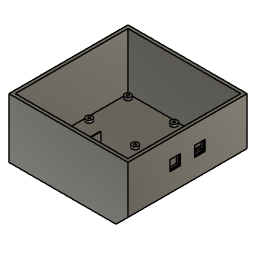
WeatherBox (Autodesk Fusion 360 design; units mm, degrees)
Autodesk Fusion 360 part; units mm, degrees
note: some values were not read from the file. Set by a fixed rule: which face or edge a step refers to.
sketch "Enclosure" plane through (0, 0, 0) normal (0, 0, 1) x (1, 0, 0)
  line L0 (0, 0) -> (150, 0)
  line L1 (150, 0) -> (150, 150)
  line L2 (150, 150) -> (0, 150)
  line L3 (0, 150) -> (0, 0)
  dimension "d1" = 150
  dimension "d2" = 150
  constraint horizontal L0
  constraint vertical L1
  constraint horizontal L2
  constraint vertical L3
  constraint coincident L0.start L3.end
  measures "d1" distance of L0.start L0.end
  measures "d2" distance of L0.start L2.end
extrude "Extrude1" add sketch "Enclosure" along normal blind 75 makes body 1
chamfer "Chamfer1" distance 15 angle 45 1 edges at (150, 75, 0) on bodies 1
shell "Shell1" thickness 4 removed faces 1 at (50, 100, 75) on bodies 1
sketch "Pi Mount" plane through (0, 0, 4) normal (0, 0, 1) x (-1, 0, 0)
  line L0 (-4, -146) -> (-4, -4)
  line L1 (-4, -4) -> (-133.3431, -4)
  line L2 (-133.3431, -146) -> (-4, -146)
  circle A0 centre (-9, -141) radius 4
  line L3 (-133.3431, -4) -> (-133.3431, -146)
  dimension "d13" = 8
  dimension "d39" = 5
  dimension "d40" = 5
  measures "d13" diameter of A0
  measures "d39" distance of L2 A0.centre
  measures "d40" distance of L0 A0.centre
extrude "Extrude2" add sketch "Pi Mount" along normal blind 3.1 contours A0 bodies 1
hole "Hole2" at (9, 141, 7.1) direction (0, 0, -1) diameter 2.9 depth 3.1 tip angle 180 bodies 1
pattern_linear "R-Pattern1" count 2 spacing 58 along (1, 0, 0) count 2 spacing 49 along (0, -1, 0) of "Extrude2", "Hole2"
sketch "Camera Holes" plane through (150, 0, 0) normal (1, 0, 0) x (0, 1, 0)
  line L0 (150, 15) -> (150, 75)
  line L1 (150, 75) -> (0, 75)
  line L2 (0, 75) -> (0, 15)
  line L3 (65, 39.45) -> (53.9, 39.45)
  line L4 (53.9, 39.45) -> (53.9, 50.55)
  line L5 (53.9, 50.55) -> (65, 50.55)
  line L6 (65, 50.55) -> (65, 39.45)
  line L7 (65, 39.45) -> (53.9, 50.55) construction
  line L8 (53.9, 39.45) -> (65, 50.55) construction
  line L9 (0, 45) -> (150, 45) construction
  line L10 (75, 75) -> (75, 0) construction
  line L11 (96.1, 39.45) -> (85, 50.55) construction
  line L12 (85, 39.45) -> (96.1, 50.55) construction
  line L13 (85, 39.45) -> (85, 50.55)
  line L14 (85, 50.55) -> (96.1, 50.55)
  line L15 (96.1, 50.55) -> (96.1, 39.45)
  line L16 (96.1, 39.45) -> (85, 39.45)
  line L17 (66, 38.45) -> (52.9, 38.45)
  line L18 (52.9, 38.45) -> (52.9, 51.55)
  line L19 (52.9, 51.55) -> (66, 51.55)
  line L20 (66, 51.55) -> (66, 38.45)
  line L21 (97.1, 38.45) -> (84, 38.45)
  line L22 (84, 38.45) -> (84, 51.55)
  line L23 (84, 51.55) -> (97.1, 51.55)
  line L24 (97.1, 51.55) -> (97.1, 38.45)
  line L25 (0, 15) -> (150, 15)
  point P0 (59.45, 45)
  point P1 (90.55, 45)
  dimension "d92" = 11.1
  dimension "d93" = 11.1
  dimension "d168" = 11.1
  dimension "d169" = 11.1
  dimension "d170" = 20
  dimension "d177" = -1
  dimension "d178" = -1
  constraint horizontal L3
  constraint perpendicular L3 L4
  constraint parallel L3 L5
  constraint parallel L4 L6
  constraint coincident L7 P0
  constraint coincident L8 P0
  constraint midpoint L2 L9.start
  constraint midpoint L0 L9.end
  constraint coincident P0 L9
  constraint midpoint L1 L10.start
  constraint horizontal L16
  constraint perpendicular L13 L16
  constraint parallel L14 L16
  constraint parallel L13 L15
  constraint coincident P1 L11
  constraint coincident P1 L12
  constraint symmetric L6 L10 L13
  constraint collinear L19 L23
  measures "d92" distance of L4.end L5.end
  measures "d93" distance of L3.end L4.end
  measures "d168" distance of L12.end L11.end
  measures "d169" distance of L12.start L11.end
  measures "d170" distance of L6 L13
extrude "Extrude6" cut sketch "Camera Holes" against normal up to surface (4 mm away) contours L3 L4 L5 L6 | L13 L14 L15 L16 bodies 1
extrude "Extrude10" cut sketch "Camera Holes" against normal blind 1.5375 contours L17 L18 L19 L20 | L21 L22 L23 L24 bodies 1
sketch "Camera Mounts" plane through (146, 0, 0) normal (-1, 0, 0) x (0, -1, 0)
  line L0 (-65, 39.45) -> (-65, 50.55)
  line L1 (-65, 50.55) -> (-53.9, 50.55)
  line L2 (-53.9, 50.55) -> (-53.9, 39.45)
  line L3 (-53.9, 39.45) -> (-65, 39.45)
  line L4 (-4, 16.6569) -> (-4, 75)
  line L5 (-4, 75) -> (-146, 75)
  line L6 (-146, 75) -> (-146, 16.6569)
  line L7 (-69.95, 57.6) -> (-48.95, 57.6) construction
  line L8 (-48.95, 57.6) -> (-48.95, 45.1) construction
  line L9 (-48.95, 45.1) -> (-69.95, 45.1) construction
  line L10 (-69.95, 45.1) -> (-69.95, 57.6) construction
  line L11 (-59.45, 50.55) -> (-59.45, 45) construction
  line L12 (-59.45, 45) -> (-53.9, 45) construction
  line L13 (-85, 39.45) -> (-96.1, 39.45)
  line L14 (-96.1, 39.45) -> (-96.1, 50.55)
  line L15 (-96.1, 50.55) -> (-85, 50.55)
  line L16 (-85, 50.55) -> (-85, 39.45)
  line L17 (-101.05, 57.6) -> (-80.05, 57.6) construction
  line L18 (-101.05, 45.1) -> (-101.05, 57.6) construction
  line L19 (-80.05, 45.1) -> (-101.05, 45.1) construction
  line L20 (-80.05, 57.6) -> (-80.05, 45.1) construction
  line L21 (-85, 45) -> (-90.55, 45) construction
  line L22 (-90.55, 45) -> (-90.55, 50.55) construction
  line L23 (-146, 16.6569) -> (-4, 16.6569)
  dimension "d131" = 21
  dimension "d132" = 12.5
  dimension "d173" = 21
  dimension "d174" = 12.5
  dimension "d176" = 0.1
  constraint horizontal L7
  constraint vertical L8
  constraint horizontal L9
  constraint vertical L10
  constraint midpoint L1 L11.start
  constraint perpendicular L1 L11
  constraint midpoint L2 L12.end
  constraint perpendicular L2 L12
  constraint horizontal L17
  constraint vertical L20
  constraint horizontal L19
  constraint vertical L18
  constraint midpoint L16 L21.start
  constraint midpoint L15 L22.end
  constraint perpendicular L15 L22
  constraint symmetric L18 L20 L22
  constraint collinear L9 L19
  measures "d131" distance of L7.start L7.end
  measures "d132" distance of L7.start L9.end
  measures "d173" distance of L17.start L17.end
  measures "d174" distance of L17.start L18.start
  measures "d176" distance of L19 L21
hole "Hole7" at (146, 48.95, 57.6) at (146, 69.95, 45.1) at (146, 80.05, 57.6) at (146, 101.05, 57.6) at (146, 101.05, 45.1) at (146, 80.05, 45.1) at (146, 69.95, 57.6) at (146, 48.95, 45.1) direction (1, 0, 0) diameter 2.9 depth 2 tip angle 180 bodies 1
sketch "Camera Posts" plane through (146, 0, 0) normal (-1, 0, 0) x (0, -1, 0)
  circle A0 centre (-101.05, 45.1) radius 1.45
  circle A1 centre (-80.05, 57.6) radius 1.45
  circle A2 centre (-48.95, 45.1) radius 1.45
  circle A3 centre (-69.95, 57.6) radius 1.45
  circle A4 centre (-48.95, 57.6) radius 1.45
  circle A5 centre (-69.95, 45.1) radius 1.45
  circle A6 centre (-101.05, 57.6) radius 1.45
  circle A7 centre (-80.05, 45.1) radius 1.45
  line L0 (-65, 39.45) -> (-65, 50.55)
  line L1 (-65, 50.55) -> (-53.9, 50.55)
  line L2 (-53.9, 50.55) -> (-53.9, 39.45)
  line L3 (-53.9, 39.45) -> (-65, 39.45)
  line L4 (-85, 39.45) -> (-96.1, 39.45)
  line L5 (-96.1, 39.45) -> (-96.1, 50.55)
  line L6 (-96.1, 50.55) -> (-85, 50.55)
  line L7 (-85, 50.55) -> (-85, 39.45)
  line L8 (-4, 16.6569) -> (-4, 75)
  line L9 (-4, 75) -> (-146, 75)
  line L10 (-146, 75) -> (-146, 16.6569)
  circle A8 centre (-101.05, 57.6) radius 3.95
  circle A9 centre (-80.05, 57.6) radius 3.95
  circle A10 centre (-101.05, 45.1) radius 3.95
  circle A11 centre (-80.05, 45.1) radius 3.95
  circle A12 centre (-69.95, 57.6) radius 3.95
  circle A13 centre (-48.95, 57.6) radius 3.95
  circle A14 centre (-48.95, 45.1) radius 3.95
  circle A15 centre (-69.95, 45.1) radius 3.95
  line L11 (-146, 16.6569) -> (-4, 16.6569)
  dimension "d193" = 2.5
  constraint equal A8 A10
  constraint equal A8 A11
  constraint equal A8 A9
  constraint equal A8 A12
  constraint equal A8 A15
  constraint equal A8 A14
  constraint equal A8 A13
extrude "Extrude11" add sketch "Camera Posts" along normal blind 7 contours A8 | A9 | A10 | A11 | A12 | A13 | A14 | A15 bodies 1
sketch "SPS30 Mount" plane through (0, 4, 0) normal (0, 1, 0) x (-1, 0, 0)
  line L0 (-4, 75) -> (-146, 75)
  line L1 (-133.3431, 4) -> (-4, 4)
  line L2 (-130, 64) -> (-82.45, 64)
  line L3 (-82.45, 64) -> (-82.45, 16.45)
  line L4 (-82.45, 16.45) -> (-130, 16.45)
  line L5 (-130, 16.45) -> (-130, 64)
  line L6 (-81.45, 15.45) -> (-131, 15.45)
  line L7 (-131, 15.45) -> (-131, 65)
  line L8 (-131, 65) -> (-81.45, 65)
  line L9 (-81.45, 65) -> (-81.45, 15.45)
  line L10 (-102.45, 16.45) -> (-102.45, 15.45)
  line L11 (-130, 16.45) -> (-130, 15.45)
  line L12 (-84.45, 64) -> (-84.45, 65)
  line L13 (-125, 64) -> (-125, 65)
  line L14 (-139.7177, 40.225) -> (-2.7177, 40.225) construction
  line L15 (-106.225, 64) -> (-106.225, 16.45) construction
  line L16 (-130, 40.225) -> (-82.45, 40.225) construction
  line L17 (-4, 4) -> (-4, 75)
  line L18 (-146, 75) -> (-146, 16.6569)
  line L19 (-99.45, 64) -> (-99.45, 75)
  line L20 (-99.45, 75) -> (-98.45, 75)
  line L21 (-98.45, 75) -> (-98.45, 64)
  line L22 (-99.45, 64) -> (-98.45, 64)
  line L23 (-77.45, 40.225) -> (-135, 40.225) construction
  circle A0 centre (-77.45, 40.225) radius 2.35
  circle A1 centre (-135, 40.225) radius 2.35
  circle A2 centre (-135, 40.225) radius 4.85
  circle A3 centre (-77.45, 40.225) radius 4.85
  line L24 (-77.45, 45.075) -> (-135, 45.075)
  line L25 (-135, 35.375) -> (-77.45, 35.375)
  line L26 (-146, 16.6569) -> (-133.3431, 4)
  dimension "d118" = 47.55
  dimension "d119" = 47.55
  dimension "d121" = -1
  dimension "d122" = 20
  dimension "d124" = 2
  dimension "d125" = 5
  dimension "d143" = 16
  dimension "d182" = 15
  dimension "d184" = 10
  dimension "d203" = 1
  dimension "d225" = 57.55
  dimension "d229" = 4.7
  dimension "d230" = 4.7
  dimension "d231" = 2.5
  dimension "d232" = 2.5
  constraint horizontal L2
  constraint vertical L3
  constraint horizontal L4
  constraint vertical L5
  constraint coincident L4 L10.start
  constraint coincident L6 L10.end
  constraint perpendicular L6 L10
  constraint coincident L6 L11.end
  constraint perpendicular L6 L11
  constraint coincident L2 L12.start
  constraint coincident L8 L12.end
  constraint perpendicular L8 L12
  constraint coincident L2 L13.start
  constraint coincident L8 L13.end
  constraint perpendicular L8 L13
  constraint midpoint L2 L15.start
  constraint midpoint L4 L15.end
  constraint midpoint L5 L16.start
  constraint midpoint L3 L16.end
  constraint collinear L14 L16
  constraint vertical L19
  constraint horizontal L20
  constraint vertical L21
  constraint coincident L0 L19.end
  constraint coincident L2 L19.start
  constraint coincident L2 L21.end
  constraint coincident L14 L23.start
  constraint perpendicular L15 L23
  constraint midpoint L15 L23
  constraint coincident L23.start A0.centre
  constraint coincident L23.end A1.centre
  constraint coincident A3 L24.start
  constraint coincident A2 L24.end
  constraint coincident A2 L25.start
  constraint coincident A3 L25.end
  constraint tangent A3 L24
  constraint tangent A3 L25
  constraint tangent A2 L25
  constraint tangent A2 L24
  measures "d118" distance of L2.start L4.end
  measures "d119" distance of L2.start L2.end
  measures "d122" distance of L3 L10
  measures "d124" distance of L3 L12
  measures "d125" distance of L5 L13
  measures "d143" distance of L3 L21
  measures "d182" distance of L7 L18
  measures "d184" distance of L0 L8
  measures "d203" distance of L21.end L19.start
  measures "d225" distance of L23.start L23.end
  measures "d229" diameter of A0
  measures "d230" diameter of A1
extrude "Extrude8" add sketch "SPS30 Mount" along normal blind 5 contours L2 L3 L8 L9 L12 L24 | L2 L5 L7 L8 L13 L24 | L9 A3 L24 | L3 L9 A3 L24 L25 | L5 L7 A2 L24 L25 | L7 A2 L24 | L9 A3 | L9 A3 | L7 A2 | L7 A2 | L9 A3 L25 | L3 L4 L6 L9 L10 L25 | L7 A2 L25 | L5 L6 L7 L11 L25 bodies 1
extrude "Extrude12" add sketch "SPS30 Mount" along normal blind 12.5 contours L0 L8 L19 L20 L21 | L2 L8 L19 L21 L22 bodies 1
sketch "AS3935 Mount" plane through (0, 0, 4) normal (0, 0, 1) x (-1, 0, 0)
  circle A0 centre (-67, -92) radius 4
  circle A1 centre (-9, -92) radius 4
  circle A2 centre (-67, -141) radius 4
  circle A3 centre (-9, -141) radius 4
  line L0 (-4, -146) -> (-4, -4)
  line L1 (-4, -4) -> (-133.3431, -4)
  line L2 (-133.3431, -146) -> (-4, -146)
  line L3 (-136, -136) -> (-110, -136) construction
  line L4 (-110, -136) -> (-110, -110) construction
  line L5 (-110, -110) -> (-136, -110) construction
  line L6 (-136, -110) -> (-136, -136) construction
  circle A4 centre (-133.25, -112.75) radius 2.35
  circle A5 centre (-133.25, -133.25) radius 2.35
  circle A6 centre (-133.25, -133.25) radius 4.85
  circle A7 centre (-133.25, -112.75) radius 4.85
  line L7 (-112.5, -136) -> (-114.5, -136)
  line L8 (-114.5, -136) -> (-114.5, -110)
  line L9 (-114.5, -110) -> (-112.5, -110)
  line L10 (-112.5, -110) -> (-112.5, -136)
  line L11 (-133.3431, -4) -> (-133.3431, -146)
  point P0 (-133.25, -133.25)
  point P1 (-133.25, -112.75)
  dimension "d211" = 26
  dimension "d212" = 26
  dimension "d213" = 2.75
  dimension "d214" = 2.75
  dimension "d215" = 2.75
  dimension "d216" = 2.75
  dimension "d217" = 4.7
  dimension "d218" = 4.7
  dimension "d219" = 2.5
  dimension "d220" = 2.5
  dimension "d223" = 2
  dimension "d224" = 2.5
  dimension "d241" = 10
  constraint horizontal L3
  constraint vertical L4
  constraint horizontal L5
  constraint vertical L6
  constraint coincident P1 A4.centre
  constraint coincident P0 A5.centre
  constraint horizontal L7
  constraint vertical L8
  constraint horizontal L9
  constraint vertical L10
  constraint coincident L5 L8.end
  constraint coincident L3 L7.start
  measures "d211" distance of L3.start L3.end
  measures "d212" distance of L3.start L5.end
  measures "d213" distance of L3 P0
  measures "d214" distance of L6 P0
  measures "d215" distance of L6 P1
  measures "d216" distance of L5 P1
  measures "d217" diameter of A4
  measures "d218" diameter of A5
  measures "d223" distance of L7.start L7.end
  measures "d224" distance of L4 L10
  measures "d241" distance of L2 L3
extrude "Extrude13" add sketch "AS3935 Mount" along normal blind 6 contours A5 A6 L11 | A5 A6 L11 | A4 A7 L11 | A4 A7 L11 | L7 L8 L9 L10 bodies 1
fillet "Fillet1" radius 0.5 8 edges at (148, 53.9, 50.55) (148, 65, 39.45) (148, 65, 50.55) (148, 53.9, 39.45) (148, 96.1, 39.45) (148, 85, 39.45) (148, 85, 50.55) (148, 96.1, 50.55) on bodies 1
sketch "Wall STEMMA Mounts" plane through (0, 4, 0) normal (0, 1, 0) x (-1, 0, 0)
  line L0 (-84.45, 64) -> (-84.45, 65)
  line L1 (-84.45, 65) -> (-81.45, 65)
  line L2 (-81.45, 65) -> (-81.45, 45.075)
  line L3 (-81.45, 45.075) -> (-77.45, 45.075)
  arc A0 (-77.45, 35.375) -> (-77.45, 45.075) centre (-77.45, 40.225) ccw
  line L4 (-77.45, 35.375) -> (-81.45, 35.375)
  line L5 (-81.45, 35.375) -> (-81.45, 15.45)
  line L6 (-81.45, 15.45) -> (-102.45, 15.45)
  line L7 (-102.45, 15.45) -> (-102.45, 16.45)
  line L8 (-102.45, 16.45) -> (-82.45, 16.45)
  line L9 (-82.45, 16.45) -> (-82.45, 64)
  line L10 (-82.45, 64) -> (-84.45, 64)
  line L11 (-99.45, 75) -> (-146, 75)
  line L12 (-98.45, 75) -> (-98.45, 64)
  line L13 (-98.45, 64) -> (-99.45, 64)
  line L14 (-99.45, 64) -> (-99.45, 75)
  line L15 (-133.3431, 4) -> (-4, 4)
  line L16 (-131, 45.075) -> (-131, 65)
  line L17 (-131, 65) -> (-125, 65)
  line L18 (-125, 65) -> (-125, 64)
  line L19 (-125, 64) -> (-130, 64)
  line L20 (-130, 64) -> (-130, 15.45)
  line L21 (-130, 15.45) -> (-131, 15.45)
  line L22 (-131, 15.45) -> (-131, 35.375)
  line L23 (-131, 35.375) -> (-135, 35.375)
  arc A1 (-135, 45.075) -> (-135, 35.375) centre (-135, 40.225) ccw
  line L24 (-135, 45.075) -> (-131, 45.075)
  circle A2 centre (-16.5, 65) radius 1.45
  circle A3 centre (-16.5, 65) radius 3.95
  line L25 (-146, 75) -> (-146, 16.6569)
  line L26 (-4, 4) -> (-4, 75)
  line L27 (-4, 75) -> (-98.45, 75)
  line L28 (-146, 16.6569) -> (-133.3431, 4)
  dimension "d284" = 2.9
  dimension "d285" = 2.5
  dimension "d287" = 10
  measures "d284" diameter of A2
  measures "d287" distance of L11 A2.centre
extrude "Extrude19" add sketch "Wall STEMMA Mounts" along normal blind 3 contours A3 bodies 1
pattern_linear "R-Pattern7" count 2 spacing 12.7 along (1, 0, 0) count 2 spacing 20.32 along (0, 0, -1) of "Extrude19"
pattern_linear "R-Pattern8" count 2 spacing 25 along (1, 0, 0) of "Extrude19", "R-Pattern7"
sketch "Sketch1" plane through (0, 9, 0) normal (0, 1, 0) x (-1, 0, 0) in component "SPS Bar"
  circle A0 centre (-135, 40.225) radius 2.35
  line L0 (-130, 15.45) -> (-130, 64)
  line L1 (-130, 64) -> (-125, 64)
  line L2 (-125, 64) -> (-125, 65)
  line L3 (-125, 65) -> (-131, 65)
  line L4 (-131, 35.375) -> (-131, 15.45)
  arc A1 (-135, 45.075) -> (-135, 35.375) centre (-135, 40.225) ccw
  line L5 (-131, 15.45) -> (-130, 15.45)
  circle A2 centre (-77.45, 40.225) radius 2.35
  line L6 (-81.45, 15.45) -> (-81.45, 35.375)
  arc A3 (-77.45, 35.375) -> (-77.45, 45.075) centre (-77.45, 40.225) ccw
  line L7 (-81.45, 65) -> (-84.45, 65)
  line L8 (-84.45, 65) -> (-84.45, 64)
  line L9 (-84.45, 64) -> (-82.45, 64)
  line L10 (-82.45, 64) -> (-82.45, 16.45)
  line L11 (-82.45, 16.45) -> (-102.45, 16.45)
  line L12 (-102.45, 16.45) -> (-102.45, 15.45)
  line L13 (-102.45, 15.45) -> (-81.45, 15.45)
  line L14 (-77.45, 45.075) -> (-135, 45.075)
  line L15 (-135, 35.375) -> (-77.45, 35.375)
  circle A4 centre (-77.45, 40.225) radius 1.5
  circle A5 centre (-135, 40.225) radius 1.5
  line L16 (-131, 45.075) -> (-135, 45.075)
  line L17 (-135, 35.375) -> (-131, 35.375)
  line L18 (-131, 65) -> (-131, 45.075)
  line L19 (-81.45, 35.375) -> (-77.45, 35.375)
  line L20 (-77.45, 45.075) -> (-81.45, 45.075)
  line L21 (-81.45, 45.075) -> (-81.45, 65)
  dimension "d269" = 3
  constraint coincident A3 L14.start
  constraint coincident A1 L14.end
  constraint tangent A3 L14
  constraint tangent A1 L14
  constraint coincident A1 L15.start
  constraint coincident A3 L15.end
  constraint tangent A1 L15
  constraint tangent A3 L15
  constraint concentric A2 A4
  constraint concentric A0 A5
  constraint equal A4 A5
  measures "d269" diameter of A4
extrude "Extrude1'" add sketch "Sketch1" along normal blind 3 separate body contours A0 | L0 A1 L14 L15 L16 L17 | L0 L10 L14 L15 | A3 L10 L14 L15 L19 L20 | A2 makes body 2 in component "SPS Bar"
sketch "Sketch2" plane through (0, 9, 0) normal (0, -1, 0) x (1, 0, 0) in component "SPS Bar"
  circle A0 centre (77.45, 40.225) radius 1.5
  circle A1 centre (135, 40.225) radius 1.5
  line L0 (77.45, 35.375) -> (135, 35.375)
  arc A2 (135, 35.375) -> (135, 45.075) centre (135, 40.225) ccw
  line L1 (135, 45.075) -> (77.45, 45.075)
  arc A3 (77.45, 45.075) -> (77.45, 35.375) centre (77.45, 40.225) ccw
  line L2 (78.8, 45.075) -> (120, 45.075)
  line L3 (120, 45.075) -> (120, 35.375)
  line L4 (120, 35.375) -> (78.8, 35.375)
  line L5 (78.8, 35.375) -> (78.8, 45.075)
  constraint horizontal L2
  constraint vertical L3
  constraint horizontal L4
  constraint vertical L5
  constraint coincident L0 L3.end
  constraint coincident L1 L2.start
sketch "Bar Height" plane through (0, 12, 0) normal (0, 1, 0) x (-1, 0, 0) in component "SPS Bar"
  circle A0 centre (-77.45, 40.225) radius 1.5
  circle A1 centre (-135, 40.225) radius 1.5
  line L0 (-135, 35.375) -> (-77.45, 35.375)
  arc A2 (-77.45, 35.375) -> (-77.45, 45.075) centre (-77.45, 40.225) ccw
  line L1 (-77.45, 45.075) -> (-135, 45.075)
  arc A3 (-135, 45.075) -> (-135, 35.375) centre (-135, 40.225) ccw
  line L2 (-82.45, 64) -> (-82.45, 16.45)
  line L3 (-130, 15.45) -> (-130, 64)
  line L4 (-80.45, 64) -> (-80.45, 22.8)
  line L5 (-132, 21.8) -> (-132, 64)
  dimension "d272" = -2
  dimension "d273" = -2
extrude "Extrude3" add sketch "Bar Height" along normal blind 12 contours L0 L1 L3 L5 | L0 L1 L2 L3 | L0 L1 L2 L4 bodies 2 in component "SPS Bar"
sketch "SPS Cut" plane through (0, 9, 0) normal (0, -1, 0) x (1, 0, 0) in component "SPS Bar"
  circle A0 centre (77.45, 40.225) radius 1.5
  circle A1 centre (135, 40.225) radius 1.5
  line L0 (77.45, 35.375) -> (135, 35.375)
  arc A2 (135, 35.375) -> (135, 45.075) centre (135, 40.225) ccw
  line L1 (135, 45.075) -> (77.45, 45.075)
  arc A3 (77.45, 45.075) -> (77.45, 35.375) centre (77.45, 40.225) ccw
  line L2 (130, 15.45) -> (130, 64)
  line L3 (82.45, 64) -> (82.45, 16.45)
extrude "Extrude4" cut sketch "SPS Cut" against normal blind 12.85 contours L0 L1 L2 L3 bodies 2 in component "SPS Bar"
fillet "Fillet1'" radius 3 4 edges at (80.45, 12, 40.225) (80.45, 24, 40.225) (132, 24, 40.225) (132, 12, 40.225) on bodies 2 in component "SPS Bar"
component "SPS Bar" placed x (1, 0, 0) y (0, 1, 0) z (0, 0, 1) at (0, 0, 0)
equation "PI_MOUNT_HOLE_SEP_W = 58 mm" comment "Distance between Pi mount holes (parallel GPIO)"
equation "PI_MOUNT_HOLE_SEP_H = 49 mm" comment "Distance between Pi mount holes (perpendicular GPIO)"
equation "d14 = PI_BOTTOM_CLEARANCE"
equation "PI_BOTTOM_CLEARANCE = 3.1 mm" comment "Height of cooler mount pins from bottom surface of Pi"
equation "d17 = PI_BOTTOM_CLEARANCE"
equation "d22 = PI_MOUNT_HOLE_SEP_W"
equation "d23 = PI_MOUNT_HOLE_SEP_H"
equation "LTR390_MOUNT_HOLE_SEP_W = 0.8 mm"
equation "LTR390_MOUNT_HOLE_SEP_H = 0.5 mm"
equation "LTR390_W = 1 mm"
equation "LTR390_H = 0.7 mm"
equation "STEMMA_W = 25.4 mm" comment "STEMMA Board Width"
equation "STEMMA_H = 17.78 mm" comment "STEMMA Board Length"
equation "STEMMA_MOUNT_HOLE_SEP_W = 20.32 mm" comment "STEMMA Mount Hole Separation Width"
equation "STEMMA_MOUNT_HOLE_SEP_H = 12.7 mm" comment "STEMMA Mount Hole Separation Length"
equation "AS3935_HOLE = 3 mm"
equation "AS3935_W = 26 mm"
equation "d92 = CAM_W + 0.2 mm"
equation "d93 = CAM_W + 0.2 mm"
equation "ARDUCAM_COVER_W = 31.5 mm"
equation "ARDUCAM_COVER_H = 30.5 mm"
equation "CAM_W = 10.9 mm"
equation "SPS30_EXHAUST_W = 14.8 mm"
equation "SPS30_EXHAUST_H = 4.75 mm"
equation "SPS30_INTAKE_W = 6.6 mm"
equation "SPS30_INTAKE_H = 3.5 mm"
equation "SPS30_W = 41.2 mm"
equation "SPS30_TOP_INTAKE_W = 10 mm"
equation "SPS30_TOP_INTAKE_H = 1.2 mm"
equation "d118 = SPS30_W + ( 0.125 in * 2 )"
equation "d119 = SPS30_W + ( 0.125 in * 2 )"
equation "AS3935_HOLE_SPACING = 30.5 mm"
equation "d168 = CAM_W + 0.2 mm"
equation "d169 = CAM_W + 0.2 mm"
equation "d179 = -CAMERA_PROTECTOR_THICKNESS + 0.05 mm"
equation "CAMERA_PROTECTOR_THICKNESS = 0.0625 in"
equation "d211 = AS3935_W"
equation "d212 = AS3935_W"
equation "d225 = d119 + 10 mm"
equation "d276 = -12.5 mm - ( 0.125 in * 2 ) + 5 mm + 1 mm"
equation "d292 = STEMMA_MOUNT_HOLE_SEP_H"
equation "d293 = -STEMMA_MOUNT_HOLE_SEP_W"
named bodies: "Enclosure"
